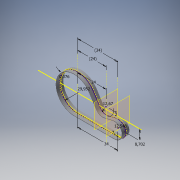
# Autodesk Inventor part: PasekZebaty
Saved by Autodesk Inventor 2019 (Build 230136000, 136)
## iProperties
Created: 2020-05-22
Part Number: PasekZebaty
Material: Generic
Document SubType Name: Modeling
Designer: estee
Density: 1 g/cm^3
Appearance: Default
Author: estee
Autodesk Inventor part; units mm, degrees
ref_plane "XZ Plane" through (0, 0, 0) normal (0, 1, 0) x (-1, 0, 0)
ref_plane "XY Plane" through (0, 0, 0) normal (0, 0, 1) x (1, 0, 0)
ref_plane "Work Plane1" through (34, 0, 0) normal (1, 0, 0) x (0, 1, 0)
ref_plane "Work Plane2" through (24, 0, 0) normal (1, 0, 0) x (0, 1, 0)
sketch "Sketch1" plane through (0, 0, 0) normal (0, 0, 1) x (1, 0, 0)
  arc A0 (12.627, 8.0522) -> (0, -14.976) centre (0, 0) ccw
  arc A1 (34, -14.976) -> (32.6451, -2.576) centre (34, -8.702) ccw
  arc A2 (18.6586, -1.4062) -> (25.3681, -4.1855) centre (24, 2) ccw
  line L0 (-33.2773, 0) -> (53.768, 0) projected
  line L1 (0, -14.976) -> (34, -14.976)
  line L2 (25.3681, -4.1855) -> (32.6451, -2.576)
  line L3 (12.627, 8.0522) -> (18.6586, -1.4062)
  line L4 (0, 28.4127) -> (0, -24.5804) construction
  line L5 (34, 28.4127) -> (34, -24.5804) construction
  line L6 (24, 28.4127) -> (24, -24.5804) construction
  arc A3 (12.9441, 8.2544) -> (0, -15.352) centre (0, 0) ccw
  line L7 (12.9441, 8.2544) -> (18.9757, -1.204)
  arc A4 (18.9757, -1.204) -> (25.2869, -3.8184) centre (24, 2) ccw
  line L8 (25.2869, -3.8184) -> (32.5639, -2.2089)
  arc A5 (34, -15.352) -> (32.5639, -2.2089) centre (34, -8.702) ccw
  line L9 (34, -15.352) -> (0, -15.352)
  dimension "d2" = 29.952
  dimension "d3" = 12.548
  dimension "d4" = 12.67
  dimension "d5" = 34
  dimension "d6" = 24
  dimension "d7" = 8.702
  dimension "d8" = 2
  dimension "d9" = 34
  dimension "d10" = 24
  dimension "d13" = 0.376
  constraints: 12 end point, 12 point on circle, 6 centre point, 5 tangent, 1 coincident, 1 point on line, 5 other
  measures "d2" diameter of A0
  measures "d3" diameter of A1
  measures "d4" diameter of A2
  measures "d5" horizontal distance of A1.centre A0.centre
  measures "d6" horizontal distance of A0.centre A2.centre
  measures "d7" distance from line of L0 A1.centre
  measures "d8" distance from line of L0 A2.centre
  measures "d9" distance between parallel lines of L5 L4
  measures "d10" distance between parallel lines of L4 L6
  measures "d13" radial gap between concentric circles of A0 A3
pattern_of_nothing "Rectangular Pattern1"
extrude "Extrusion1" add sketch "Sketch1" along normal mid plane 6 contours A0 L0 A3 L7 L3 | A0 L1 A1 L2 A2 L3 L0 L7 A4 L8 A5 L9 A3
equation "\"start1\" = d9"
equation "\"start2\" = d10"
body "Solid1"
